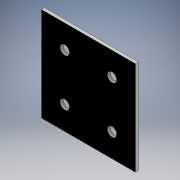
# Autodesk Inventor part: 00_LED-ARRAY_4x4
Saved by Autodesk Inventor 2019 (Build 230136000, 136)
## iProperties
Created: 2020-11-27
Part Number: 00_LED-ARRAY_4x4
Material: Generic
Document SubType Name: Modeling
Designer: UC2
Density: 1 g/cm^3
Appearance: Default
Author: UC2
Autodesk Inventor part; units mm, degrees
ref_plane "YZ Plane" through (0, 0, 0) normal (1, 0, 0) x (0, 1, 0)
ref_plane "XZ Plane" through (0, 0, 0) normal (0, 1, 0) x (-1, 0, 0)
ref_plane "XY Plane" through (0, 0, 0) normal (0, 0, 1) x (1, 0, 0)
sketch "Skizze1" plane through (0, 0, 0) normal (0, 0, 1) x (1, 0, 0)
  line L0 (-15, -15) -> (15, -15)
  line L1 (15, -15) -> (15, 15)
  line L2 (15, 15) -> (-15, 15)
  line L3 (-15, 15) -> (-15, -15)
  line L4 (-15, -15) -> (15, 15) construction
  line L5 (15, -15) -> (-15, 15) construction
  point P0 (0, 0)
  dimension "d0" = 30
  dimension "d1" = 30
  constraints: 12 end point, 2 midpoint, 2 parallel, 1 horizontal, 1 perpendicular
  measures "d0" distance of L1.end L2.end
  measures "d1" distance of L0.end L1.end
extrude "Extrusion1" add sketch "Skizze1" along normal blind 1
sketch "Sketch2" plane through (0, 0, 1) normal (0, 0, 1) x (1, 0, 0)
  line L0 (-15, -15) -> (15, -15) construction
  line L1 (15, -15) -> (15, 15) construction
  line L2 (15, 15) -> (-15, 15) construction
  line L3 (-15, 15) -> (-15, -15) construction
  line L4 (-7.535, 7.535) -> (7.535, 7.535) construction
  line L5 (7.535, 7.535) -> (7.535, -7.535) construction
  line L6 (7.535, -7.535) -> (-7.535, -7.535) construction
  line L7 (-7.535, -7.535) -> (-7.535, 7.535) construction
  point P0 (0, 0)
  dimension "d4" = 7.465
  constraints: 8 end point, 3 other
  measures "d4" distance between parallel lines of L2 L4
hole "Hole1" at (-7.535, 7.535, 1) at (7.535, 7.535, 1) at (7.535, -7.535, 1) at (-7.535, -7.535, 1) direction (0, 0, -1) diameter 2.93 end through all
equation "\"d1\" = d0"
